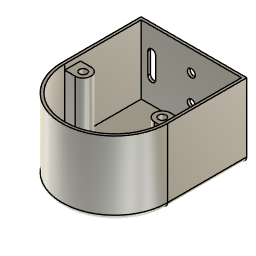
TRARM02_Link4B_30x40x28 (Autodesk Fusion 360 design; units mm, degrees)
Autodesk Fusion 360 part; units mm, degrees
note: some values were not read from the file. Set by a fixed rule: which sketch regions a step uses.
sketch "스케치1" plane through (0, 0, 0) normal (0, 0, 1) x (1, 0, 0)
  line L0 (20, 30) -> (20, 0)
  line L1 (-20, 30) -> (-20, 0)
  arc A0 (-20, 0) -> (20, 0) centre (0, 0) ccw
  line L2 (-20, 30) -> (20, 30)
  dimension "d1" = 40
  dimension "d144" = 30
  constraint coincident A0.centre origin
  constraint tangent L0 A0
  constraint vertical L0
  constraint parallel L0 L1
  constraint horizontal L0.start L1.start
  measures "d1" diameter of A0
  measures "d144" vertical distance of A0.centre L1.start
extrude "돌출1" add sketch "스케치1" along normal blind 2
sketch "스케치14" plane through (0, 0, 2) normal (0, 0, 1) x (-1, 0, 0)
  line L0 (20, -30) -> (20, 0)
  line L1 (-20, 0) -> (-20, -30)
  arc A0 (20, 0) -> (-20, 0) centre (0, 0) ccw
  arc A1 (19, 0) -> (-19, 0) centre (0, 0) ccw
  line L2 (15, -6) -> (19, -6)
  line L3 (15, 0) -> (19, 0)
  arc A2 (15, 0) -> (15, -6) centre (15, -3) ccw
  line L4 (-15, -6) -> (-19, -6)
  arc A3 (-15, -6) -> (-15, 0) centre (-15, -3) ccw
  line L5 (19, -29) -> (19, -6)
  line L6 (-19, -6) -> (-19, -29)
  line L7 (-15, 0) -> (-19, 0)
  line L8 (-20, -30) -> (20, -30)
  line L9 (20, -30) -> (-20, -30)
  line L10 (19, -29) -> (-19, -29)
  dimension "d111" = 15
  dimension "d112" = 6
  dimension "d114" = 3
  dimension "d132" = 4
  dimension "d133" = 4
  dimension "d134" = 4
  dimension "d135" = 1
  dimension "d136" = 4
  dimension "d142" = 1
  dimension "d143" = 19
  dimension "d145" = 1
  constraint concentric A0 A1
  constraint equal A2 A3
  constraint horizontal A2.centre A3.centre
  constraint horizontal L7
  constraint vertical L6
  constraint horizontal L4
  constraint vertical L5
  constraint horizontal L3
  constraint coincident A1.start L3.end
  constraint horizontal L2
  constraint coincident L0.start L8.end
  constraint coincident L1.end L8.start
  constraint horizontal L10
  measures "d111" horizontal distance of A0.centre A2.centre
  measures "d112" diameter of A2
  measures "d114" vertical distance of A0.centre A2.centre
  measures "d132" distance of L3.start A1.start
  measures "d133" distance of L2.start L2.end
  measures "d134" distance of A1.end A3.end
  measures "d135" distance of L1 L6
  measures "d136" distance of L4.start L4.end
  measures "d142" distance of L0 L5
  measures "d143" radius of A1
  measures "d145" distance of L9 L10
extrude "돌출18" add sketch "스케치14" along normal blind 26
sketch "스케치17" plane through (0, 0, 28) normal (0, 0, 1) x (-1, 0, 0)
  line L0 (-19, -6) -> (-15, -6)
  line L1 (-15, 0) -> (-19, 0)
  arc A0 (-15, -6) -> (-15, 0) centre (-15, -3) ccw
  arc A1 (15, 0) -> (15, -6) centre (15, -3) ccw
  line L2 (19, 0) -> (15, 0)
  line L3 (15, -6) -> (19, -6)
  line L4 (19, -6) -> (19, 0)
  line L5 (-19, -6) -> (-19, 0)
  point P0 (15, 0)
  constraint coincident L3.end L4.start
  constraint coincident L2.start L4.end
  constraint coincident L0.start L5.start
  constraint coincident L1.end L5.end
extrude "돌출19" cut sketch "스케치17" against normal blind 2
sketch "스케치18" plane through (0, 0, 26) normal (0, 0, 1) x (-1, 0, 0)
  circle A0 centre (15, -3) radius 1.45
  arc A1 (15, 0) -> (15, -6) centre (15, -3) ccw
  circle A2 centre (-15, -3) radius 1.45
  arc A3 (-15, -6) -> (-15, 0) centre (-15, -3) ccw
  constraint concentric A0 A1
  constraint equal A0 A2
extrude "돌출20" cut sketch "스케치18" against normal blind 5
fillet "필렛4" radius 2 3 edges at (20, 15, 0) (0, -20, 0) (-20, 15, 0)
sketch "스케치21" plane through (0, 30, 0) normal (0, 1, 0) x (-1, 0, 0)
  circle A0 centre (0, 10) radius 1.5
  circle A1 centre (0, 20) radius 1.5
  dimension "d153" = 3
  dimension "d159" = 10
  dimension "d160" = 10
  constraint vertical origin A0.centre
  constraint equal A0 A1
  constraint vertical origin A1.centre
  measures "d153" diameter of A0
  measures "d159" distance of origin A0.centre
  measures "d160" distance of A0.centre A1.centre
extrude "돌출23" cut sketch "스케치21" against normal blind 1
sketch "스케치22" plane through (0, 30, 0) normal (0, 1, 0) x (-1, 0, 0)
  line L0 (-16.5, 11) -> (-16.5, 19)
  line L1 (-13.5, 11) -> (-13.5, 19)
  arc A0 (-16.5, 11) -> (-13.5, 11) centre (-15, 11) ccw
  arc A1 (-13.5, 19) -> (-16.5, 19) centre (-15, 19) ccw
  line L2 (13.5, 11) -> (13.5, 19)
  arc A2 (16.5, 19) -> (13.5, 19) centre (15, 19) ccw
  line L3 (16.5, 11) -> (16.5, 19)
  arc A3 (13.5, 11) -> (16.5, 11) centre (15, 11) ccw
  dimension "d161" = 8
  dimension "d162" = 1.5
  dimension "d163" = 15
  dimension "d164" = 11
  dimension "d167" = 8
  dimension "d168" = 1.5
  dimension "d169" = 15
  constraint tangent L1 A1
  constraint parallel L0 L1
  constraint equal A0 A1
  constraint tangent L0 A0
  constraint tangent L0 A1
  constraint vertical A0.centre A1.centre
  constraint tangent A2 L3
  constraint parallel L2 L3
  constraint equal A2 A3
  constraint tangent L2 A3
  constraint tangent L2 A2
  constraint vertical A3.centre A2.centre
  constraint horizontal A0.centre A3.centre
  measures "d161" distance of A0.centre A1.centre
  measures "d162" radius of A1
  measures "d163" horizontal distance of origin A0.centre
  measures "d164" vertical distance of origin A0.centre
  measures "d167" distance of A3.centre A2.centre
  measures "d168" radius of A2
  measures "d169" horizontal distance of origin A3.centre
extrude "돌출24" cut sketch "스케치22" against normal blind 2
